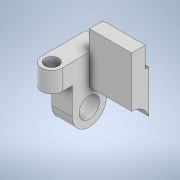
# Autodesk Inventor part: Battery_short_holder
Saved by Autodesk Inventor 2022 (Build 260153000, 153)
## iProperties
Created: 2023-01-30
Part Number: Battery_short_holder
Material: Generic
Document SubType Name: Modeling
Designer: scott
Density: 1 g/cm^3
Appearance: Default
Author: scott
Autodesk Inventor part; units mm, degrees
ref_plane "YZ Plane" through (0, 0, 0) normal (1, 0, 0) x (0, 1, 0)
ref_plane "XZ Plane" through (0, 0, 0) normal (0, 1, 0) x (-1, 0, 0)
ref_plane "XY Plane" through (0, 0, 0) normal (0, 0, 1) x (1, 0, 0)
sketch "Sketch1" plane through (0, 0, 0) normal (0, 1, 0) x (-1, 0, 0)
  circle A0 centre (7.7, 2.5) radius 1
  circle A1 centre (7.7, 2.5) radius 1.5
  line L0 (9.2, 4) -> (0, 4)
  line L1 (0, 4) -> (0, -4)
  line L2 (0, -4) -> (9.2, -4)
  line L3 (9.2, -4) -> (9.2, 4)
  line L4 (9.2, -4) -> (0, -4)
  line L5 (0, -4) -> (0, -1.5)
  line L6 (0, -1.5) -> (9.2, -1.5)
  line L7 (9.2, -1.5) -> (9.2, -4)
  line L8 (6.2, 2.5) -> (9.2, 2.5)
  line L9 (9.2, 2.5) -> (9.2, -1.5)
  line L10 (9.2, -1.5) -> (6.2, -1.5)
  line L11 (6.2, -1.5) -> (6.2, 2.5)
  point P0 (0, 0)
  point P1 (9.2, 2.5)
  dimension "d5" = 3
  dimension "d4" = 2
  dimension "d8" = 8
  dimension "d9" = 4
  dimension "d10" = 1.5
  dimension "d11" = 1.5
  dimension "d12" = 2.5
  constraints: 24 end point, 6 parallel, 3 horizontal, 3 perpendicular, 1 centre point, 1 coincident, 1 point on line, 3 other
  measures "d4" diameter of A0
  measures "d8" distance of L1.end L0.end
  measures "d9" distance from line of L2 point (0, 0)
  measures "d10" distance from line of L3 A0.centre
  measures "d11" distance from line of L0 A0.centre
  measures "d12" distance of L4.end L5.end
extrude "Extrusion1" add sketch "Sketch1" along normal blind 3 contours L8 A1 A0 | A0 L8 A1 | L3 L6 L11 A1 | L3 L2 L1 L6
sketch "Sketch2" plane through (0, 3, 0) normal (0, 1, 0) x (1, 0, 0)
  line L0 (-6.2, 1.5) -> (0, 1.5) projected
  line L1 (0, 1.5) -> (-6.2, 1.5)
  line L2 (-6.2, 1.5) -> (-6.2, 3.5)
  line L3 (-6.2, 3.5) -> (0, 3.5)
  line L4 (0, 3.5) -> (0, 1.5)
  circle A0 centre (-5.7, 3) radius 0.5
  point P0 (0, 0)
  point P1 (-6.2, 3)
  point P2 (-5.7, 3.5)
  dimension "d15" = 2
  dimension "d16" = 1
  dimension "d17" = 0.5
  constraints: 8 end point, 2 parallel, 1 centre point, 1 horizontal, 1 perpendicular, 1 tangent
  measures "d15" distance of L1.end L2.end
  measures "d16" diameter of A0
  measures "d17" distance from line of L2 A0.centre
extrude "Extrusion2" add sketch "Sketch2" along normal blind 3 contours L2 A0 L3 L4 L0 | A0
sketch "Sketch3" plane through (-9.2, 0, -4) normal (-1, 0, 0) x (0, 0, 1)
  circle A0 centre (2.5, -4) radius 2.5
  circle A1 centre (2.5, -4) radius 1.5
  line L0 (0, 0) -> (0, 3) projected
  line L1 (0, 0) -> (6.5, 0) projected
  line L2 (5, -4) -> (0, -4)
  line L3 (0, -4) -> (0, 0)
  line L4 (0, 0) -> (5, 0)
  line L5 (5, 0) -> (5, -4)
  point P0 (4, 0)
  dimension "d20" = 5
  dimension "d21" = 3
  dimension "d22" = 2.5
  dimension "d23" = 4
  constraints: 8 end point, 2 parallel, 1 centre point, 1 coincident, 1 horizontal, 1 perpendicular, 3 other
  measures "d21" diameter of A1
  measures "d22" distance from line of L0 point (2.5, -4)
  measures "d23" distance from line of L1 point (2.5, -4)
extrude "Extrusion3" add sketch "Sketch3" against normal blind 3 contours L2 A1 A0 | A0 L2 A1 | A0 L3 L1 L5
sketch "Sketch4" plane through (-6.2, 0, 2.5) normal (1, 0, 0) x (0, 0, -1)
  circle A0 centre (4, -4) radius 1.5 projected
  circle A1 centre (4, -4) radius 2.6
  line L0 (6.5, -4) -> (6.5, 0) projected
  line L1 (6.5, 0) -> (4, 0)
  line L2 (4, 0) -> (4, -4)
  line L3 (4, -4) -> (6.5, -4)
  line L4 (6.5, -4) -> (6.5, 0)
  point P0 (2.5, 0)
  point P1 (4, -1.4)
  point P2 (6.5, -3.2859)
  dimension "d26" = 5.2
  constraints: 8 end point, 2 parallel, 1 centre point, 1 coincident, 1 horizontal, 1 perpendicular
  measures "d26" diameter of A1
extrude "Extrusion4" add sketch "Sketch4" along normal up to surface (6.2 mm away) contours L2 L1 L0 A1
equation "\"d22\" = 0.5 * d20"
body "Solid1"
